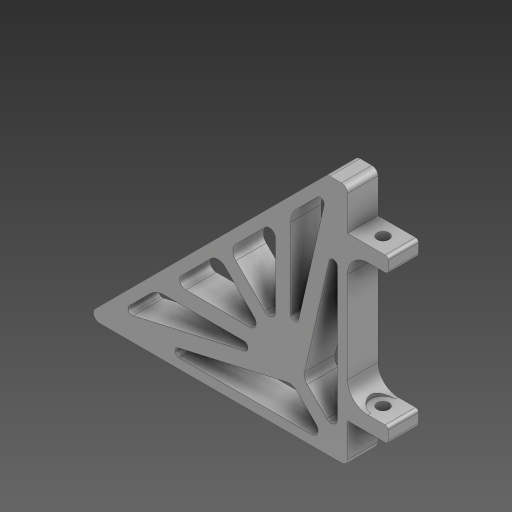
# Autodesk Inventor part: Controls Mid Support V2
Saved by Autodesk Inventor 2024 (Build 280153000, 153)
## iProperties
Created: 2023-08-31
Part Number: Controls Mid Support V2
Material: ABS Plastic
Document SubType Name: Modeling
Designer: mxs6493
Density: 1.06 g/cm^3
Appearance: Anodized - Light Gray
Mass: 80.8279 g
Surface Area: 288.648 cm^2
Volume: 76.2528 cm^3
Author: mxs6493
Autodesk Inventor part; units mm, degrees
ref_plane "YZ Plane" through (0, 0, 0) normal (1, 0, 0) x (0, 1, 0)
ref_plane "XZ Plane" through (0, 0, 0) normal (0, 1, 0) x (-1, 0, 0)
ref_plane "XY Plane" through (0, 0, 0) normal (0, 0, 1) x (1, 0, 0)
sketch "Sketch1" plane through (0, 0, 0) normal (0, 0, 1) x (1, 0, 0)
  line L0 (0, 119.501) -> (-30, 119.501)
  line L1 (-30, 119.501) -> (-32.8284, 116.6726)
  line L2 (-32.8284, 116.6726) -> (-149.501, 0)
  line L3 (0, -23.9002) -> (0, 143.4013) projected
  line L4 (0, 119.501) -> (0, 0)
  line L5 (-149.501, 0) -> (0, 0)
  line L6 (-20, 119.501) -> (-20, 0)
  line L7 (-20, 99.501) -> (0, 99.501)
  line L8 (-20, 19.501) -> (0, 19.501)
  line L9 (-20, 92.001) -> (0, 92.001)
  line L10 (-20, 27.001) -> (0, 27.001)
  point P0 (0, 27.001)
  point P1 (0, 92.001)
  point P2 (0, 99.501)
  dimension "d3" = 30
  dimension "d41" = 4
  dimension "d42" = 165
  dimension "d43" = 45
  dimension "d173" = 20
  dimension "d174" = 20
  dimension "d175" = 80
  dimension "d176" = 7.5
  dimension "d177" = 7.5
  constraints: 20 end point, 11 point on line, 5 perpendicular, 2 horizontal, 1 collinear
  measures "d3" distance of L0.start L0.end
  measures "d41" distance of L0.end L1.end
  measures "d42" distance of L1.end L2.end
  measures "d43" angle of L3 L2
  measures "d173" distance between parallel lines of L3 L6
  measures "d174" distance between parallel lines of L0 L7
  measures "d175" distance between parallel lines of L8 L7
  measures "d176" distance between parallel lines of L7 L9
  measures "d177" distance between parallel lines of L10 L8
extrude "Extrusion3" add sketch "Sketch1" along normal mid plane 15 contours L6 L5 L2 L1 L0 | L3 L9 L6 L7 | L3 L8 L6 L10
fillet "Fillet2" radius 3 2 edges at (-149.501, 0, 0) (-30, 119.501, 0)
sketch "Sketch7" plane through (0, 0, -7.5) normal (0, 0, -1) x (-1, 0, 0)
  line L0 (20, 119.501) -> (28.7574, 119.501) projected
  arc A0 (30.8787, 118.6224) -> (28.7574, 119.501) centre (28.7574, 116.501) ccw projected
  line L1 (30.8787, 118.6224) -> (144.3797, 5.1213) projected
  arc A1 (142.2584, 0) -> (144.3797, 5.1213) centre (142.2584, 3) ccw projected
  line L2 (142.2584, 0) -> (20, 0) projected
  line L3 (137.43, 5) -> (27.9289, 114.501)
  line L4 (27.9289, 114.501) -> (20, 114.501)
  line L5 (20, 5) -> (137.43, 5)
  line L6 (20, 119.501) -> (20, 0)
  line L7 (30.3033, 5) -> (83.8666, 58.5633)
  line L8 (78.5633, 63.8666) -> (20, 5.3033)
  line L9 (53.3373, 28.034) -> (132.4465, 9.9835)
  line L10 (120.5726, 5) -> (47.0737, 21.7704)
  line L11 (60.8373, 35.534) -> (106.896, 35.534)
  line L12 (114.396, 28.034) -> (53.3373, 28.034)
  line L13 (25, 114.501) -> (25, 5)
  line L14 (25, 5) -> (110.8696, 90.8696) construction
  line L15 (48.034, 33.3373) -> (29.9835, 112.4465)
  line L16 (25, 100.5726) -> (41.7704, 27.0737)
  line L17 (55.534, 40.8373) -> (55.534, 86.896)
  line L18 (48.034, 94.396) -> (48.034, 33.3373)
  line L19 (20, 0) -> (20, 19.501) projected
  line L20 (20, 19.501) -> (0, 19.501) projected
  line L21 (0, 19.501) -> (0, 27.001) projected
  line L22 (0, 27.001) -> (20, 27.001) projected
  line L23 (20, 27.001) -> (20, 92.001) projected
  line L24 (20, 92.001) -> (0, 92.001) projected
  line L25 (0, 92.001) -> (0, 99.501) projected
  line L26 (0, 99.501) -> (20, 99.501) projected
  line L27 (20, 99.501) -> (20, 119.501) projected
  point P0 (0, 0)
  point P1 (57.667, 27.0945)
  point P2 (55.3752, 24.3268)
  point P3 (25, 10.3033)
  point P4 (25, 8.4645)
  point P5 (21.4645, 5)
  point P6 (56.9274, 31.6241)
  point P7 (47.0737, 21.7704)
  point P8 (25, 100.5726)
  point P9 (41.7704, 27.0737)
  point P10 (55.534, 40.8373)
  point P11 (55.534, 86.896)
  point P12 (48.034, 33.3373)
  point P13 (29.9835, 112.4465)
  point P14 (48.034, 94.396)
  point P15 (27.5, 118.4655)
  point P16 (48.034, 33.3373)
  point P17 (48.034, 33.3373)
  dimension "d57" = 5
  dimension "d61" = 7.5
  dimension "d63" = 7.5
  dimension "d66" = 3.75
  dimension "d67" = 7.5
  dimension "d70" = 5
  dimension "d75" = 3.75
  constraints: 34 end point, 15 point on line, 8 symmetric about line, 4 parallel, 2 vertical, 1 horizontal, 1 perpendicular
  measures "d57" distance between parallel lines of L1 L3
  measures "d61" distance between parallel lines of L8 L7
  measures "d63" distance between parallel lines of L10 L9
  measures "d66" distance from line of L10 L3.start
  measures "d67" distance between parallel lines of L11 L12
  measures "d70" distance between parallel lines of L6 L13
  measures "d75" distance from line of L13.end L8
extrude "Extrusion6" cut sketch "Sketch7" against normal through all contours L16 L8 L13 | L3 L18 L15 | L3 L8 L17 | L7 L10 L5 | L3 L11 L7 | L12 L3 L9
fillet "Fillet28" radius 2 6 edges at (-53.3373, 28.034, 0) (-48.034, 33.3373, 0) (-25, 100.5726, 0) (-120.5726, 5, 0) (-132.4465, 9.9835, 0) (-29.9835, 112.4465, 0)
fillet "Fillet29" radius 10 2 edges at (-48.034, 94.396, 0) (-114.396, 28.034, 0)
fillet "Fillet30" radius 5 2 edges at (-83.8666, 58.5633, 0) (-78.5633, 63.8666, 0)
fillet "Fillet31" radius 3 6 edges at (-25, 10.3033, 0) (-30.3033, 5, 0) (-106.896, 35.534, 0) (-60.8373, 35.534, 0) (-55.534, 86.896, 0) (-55.534, 40.8373, 0)
fillet "Fillet32" radius 5 2 edges at (-41.7704, 27.0737, 0) (-47.0737, 21.7704, 0)
fillet "Fillet33" radius 3 2 edges at (-20, 119.501, 0) (-20, 0, 0)
fillet "Fillet34" radius 10 2 edges at (-20, 92.001, 0) (-20, 27.001, 0)
sketch "Sketch16" plane through (0, 92.001, -7.5) normal (0, -1, 0) x (1, 0, 0)
  line L0 (0, 0) -> (-10, 0) projected
  line L1 (-10, 0) -> (-10, 15) projected
  point P0 (0, 7.5)
  point P1 (-10, 7.5)
  dimension "d192" = 7.5
  constraints: 1 midpoint
  measures "d192" distance from line of L0 point (-10, 7.5)
hole "Hole7" at (-10, 92.001, 0) direction (0, 1, 0) diameter 5.8 end through all clearance for "Socket Head Cap Screw" size "M5" standard "Ansi Metric M Profile"
sketch "Sketch18" plane through (0, 27.001, 7.5) normal (0, 1, 0) x (1, 0, 0)
  line L0 (-10, 15) -> (0, 15) projected
  line L1 (-10, 0) -> (-10, 15) projected
  point P0 (0, 7.5)
  point P1 (-10, 7.5)
  dimension "d203" = 7.5
  constraints: 1 midpoint
  measures "d203" distance from line of L0 point (-10, 7.5)
hole "Hole8" at (-10, 27.001, 0) direction (0, -1, 0) diameter 5.8 end through all clearance for "Socket Head Cap Screw" size "M5" standard "Ansi Metric M Profile"
sketch "Sketch19" plane through (0, 27.001, 7.5) normal (0, 1, 0) x (1, 0, 0)
  line L0 (-10, 4.6) -> (-10, 10.4) projected
  circle A0 centre (-10, 7.5) radius 6
  point P0 (0, 7.5)
  dimension "d204" = 12
  constraints: 1 centre point, 1 midpoint
  measures "d204" diameter of A0
extrude "Extrusion12" cut sketch "Sketch19" along normal up to surface (65 mm away)
fillet "Fillet35" radius 1.5 4 edges at (0, 19.501, 0) (0, 27.001, 0) (0, 92.001, 0) (0, 99.501, 0)
body "Solid2"
